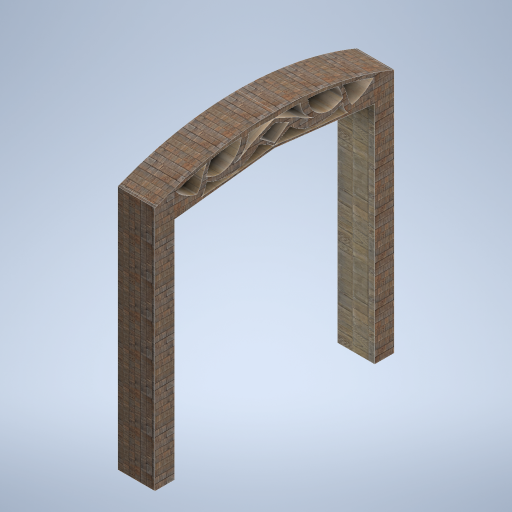
# Autodesk Inventor part: side_door_frame
Saved by Autodesk Inventor 2024.2 (Build 282272000, 272)
## iProperties
Created: 2024-05-27
Part Number: side_door_frame
Material: Wood (Maple)
Document SubType Name: Modeling
Designer: LOSTER_1
Density: 0.67 g/cm^3
Appearance: Natural Maple - Glossy Dark Tint
Author: LOSTER_1
Autodesk Inventor part; units mm, degrees
ref_plane "YZ Plane" through (0, 0, 0) normal (1, 0, 0) x (0, 1, 0)
ref_plane "XZ Plane" through (0, 0, 0) normal (0, 1, 0) x (-1, 0, 0)
ref_plane "XY Plane" through (0, 0, 0) normal (0, 0, 1) x (1, 0, 0)
sketch "Sketch1" plane through (0, 0, 0) normal (1, 0, 0) x (0, 1, 0)
  arc A0 (1227.0996, 1213.6257) -> (1219.0039, 1233.4807) centre (-1740.0857, 15.3721) ccw
  arc A1 (1293.746, 1033.6257) -> (1227.0996, 1213.6257) centre (-1739.133, 13.0159) ccw
  arc A2 (1300.346, 1013.7992) -> (1293.746, 1033.6257) centre (-1739.133, 13.0159) ccw
  arc A3 (1353.8129, 833.7992) -> (1300.346, 1013.7992) centre (-1739.133, 13.0159) ccw
  arc A4 (1359.0618, 813.7583) -> (1353.8129, 833.7992) centre (-1739.133, 13.0159) ccw
  arc A5 (1400.0832, 633.7583) -> (1359.0618, 813.7583) centre (-1739.133, 13.0159) ccw
  arc A6 (1403.9797, 613.7174) -> (1400.0832, 633.7583) centre (-1739.133, 13.0159) ccw
  arc A7 (1433.0918, 433.7174) -> (1403.9797, 613.7174) centre (-1739.133, 13.0159) ccw
  arc A8 (1453.264, 233.4731) -> (1435.7109, 413.4731) centre (-1739.133, 13.0159) ccw
  arc A9 (1435.7109, 413.4731) -> (1433.0918, 433.7174) centre (-1739.133, 13.0159) ccw
  arc A10 (1454.5841, 213.442) -> (1453.264, 233.4731) centre (-1739.133, 13.0159) ccw
  arc A11 (1460.8042, 33.0557) -> (1454.5841, 213.442) centre (-1739.133, 13.0159) ccw
  arc A12 (1460.867, 13.0444) -> (1460.8042, 33.0557) centre (-1739.133, 13.0159) ccw
  line L0 (-1280.9961, 1233.4807) -> (1219.0039, 1233.4807)
  line L1 (-1280.9961, 1233.4807) -> (-1280.9961, 1033.4807)
  line L2 (-1280.9961, 1033.4807) -> (1019.0039, 1033.4807)
  line L3 (1019.0039, 1033.4807) -> (1138.5556, 13.0444)
  line L4 (1460.867, 13.0444) -> (1469.3401, 13.0444)
  line L5 (1402.0541, 13.0444) -> (1293.7527, 249.1451)
  line L6 (1293.7527, 249.1451) -> (1163.5573, 13.0444)
  arc A13 (1208.0697, 415.2091) -> (1293.7527, 249.1451) centre (1799.1105, 615.028) ccw
  arc A14 (1232.0349, 708.2436) -> (1190.1135, 593.1028) centre (1522.2816, 537.3662) ccw
  arc A15 (1128.8881, 470.6135) -> (1251.1701, 171.9244) centre (1578.7407, 480.4058) ccw
  arc A16 (1191.7037, 709.8957) -> (1128.8881, 470.6135) centre (1578.7407, 480.4058) ccw
  arc A17 (1042.3948, 833.8278) -> (1191.7037, 709.8957) centre (1193.4877, 863.9522) ccw
  arc A18 (1400.0832, 633.7583) -> (1232.0349, 708.2436) centre (1155.9138, 309.6924) ccw
  arc A19 (1390.4476, 680.6424) -> (1228.9697, 753.7281) centre (1125.8269, 310.9107) ccw
  arc A20 (1190.1135, 593.1028) -> (1442.5544, 354.8708) centre (1416.5041, 580.1314) ccw
  arc A21 (1208.0697, 415.2091) -> (1449.7856, 279.0945) centre (1417.3067, 504.0976) ccw
  arc A22 (1290.1375, 1044.287) -> (1125.8335, 802.5328) centre (1497.6402, 726.5511) ccw
  arc A23 (1260.8526, 1126.6075) -> (1078.7798, 848.8845) centre (1573.2668, 723.2474) ccw
  arc A24 (1028.8129, 949.7563) -> (1078.7798, 848.8845) centre (1290.1521, 1016.3994) ccw
  arc A25 (1125.8335, 802.5328) -> (1228.9697, 753.7281) centre (1290.1521, 1016.3994) ccw
  line L7 (1359.0618, 13.0444) -> (1293.7527, 162.4218)
  line L8 (1293.7527, 162.4218) -> (1183.7754, 13.0444)
  line L9 (1460.867, 13.0444) -> (1635.1821, 13.0444)
  arc A26 (1219.0039, -1207.3919) -> (1227.0996, -1187.5369) centre (-1740.0857, 10.7167) ccw
  arc A27 (1227.0996, -1187.5369) -> (1293.746, -1007.5369) centre (-1739.133, 13.073) ccw
  arc A28 (1293.746, -1007.5369) -> (1300.346, -987.7104) centre (-1739.133, 13.073) ccw
  arc A29 (1300.346, -987.7104) -> (1353.8129, -807.7104) centre (-1739.133, 13.073) ccw
  arc A30 (1353.8129, -807.7104) -> (1359.0618, -787.6695) centre (-1739.133, 13.073) ccw
  arc A31 (1359.0618, -787.6695) -> (1400.0832, -607.6695) centre (-1739.133, 13.073) ccw
  arc A32 (1400.0832, -607.6695) -> (1403.9797, -587.6286) centre (-1739.133, 13.073) ccw
  arc A33 (1403.9797, -587.6286) -> (1433.0918, -407.6286) centre (-1739.133, 13.073) ccw
  arc A34 (1435.7109, -387.3843) -> (1453.264, -207.3843) centre (-1739.133, 13.073) ccw
  arc A35 (1433.0918, -407.6286) -> (1435.7109, -387.3843) centre (-1739.133, 13.073) ccw
  arc A36 (1453.264, -207.3843) -> (1454.5841, -187.3532) centre (-1739.133, 13.073) ccw
  arc A37 (1454.5841, -187.3532) -> (1460.8042, -6.9669) centre (-1739.133, 13.073) ccw
  arc A38 (1460.8042, -6.9669) -> (1460.867, 13.0444) centre (-1739.133, 13.073) ccw
  line L10 (-1280.9961, -1207.3919) -> (1219.0039, -1207.3919)
  line L11 (-1280.9961, -1207.3919) -> (-1280.9961, -1007.3919)
  line L12 (-1280.9961, -1007.3919) -> (1019.0039, -1007.3919)
  line L13 (1019.0039, -1007.3919) -> (1138.5556, 13.0444)
  line L14 (1402.0541, 13.0444) -> (1293.7527, -223.0563)
  line L15 (1293.7527, -223.0563) -> (1163.5573, 13.0444)
  arc A39 (1293.7527, -223.0563) -> (1208.0697, -389.1203) centre (1799.1105, -588.9392) ccw
  arc A40 (1190.1135, -567.014) -> (1232.0349, -682.1547) centre (1522.2816, -511.2774) ccw
  arc A41 (1251.1701, -145.8356) -> (1128.8881, -444.5247) centre (1578.7407, -454.317) ccw
  arc A42 (1128.8881, -444.5247) -> (1191.7037, -683.8069) centre (1578.7407, -454.317) ccw
  arc A43 (1191.7037, -683.8069) -> (1042.3948, -807.7389) centre (1193.4877, -837.8633) ccw
  arc A44 (1232.0349, -682.1547) -> (1400.0832, -607.6695) centre (1155.9138, -283.6036) ccw
  arc A45 (1228.9697, -727.6392) -> (1390.4476, -654.5536) centre (1125.8269, -284.8219) ccw
  arc A46 (1442.5544, -328.782) -> (1190.1135, -567.014) centre (1416.5041, -554.0426) ccw
  arc A47 (1449.7856, -253.0056) -> (1208.0697, -389.1203) centre (1417.3067, -478.0088) ccw
  arc A48 (1125.8335, -776.444) -> (1290.1375, -1018.1981) centre (1497.6402, -700.4623) ccw
  arc A49 (1078.7798, -822.7957) -> (1260.8526, -1100.5187) centre (1573.2668, -697.1585) ccw
  arc A50 (1078.7798, -822.7957) -> (1028.8129, -923.6674) centre (1290.1521, -990.3106) ccw
  arc A51 (1228.9697, -727.6392) -> (1125.8335, -776.444) centre (1290.1521, -990.3106) ccw
  line L16 (1359.0618, 13.0444) -> (1293.7527, -136.333)
  line L17 (1293.7527, -136.333) -> (1183.7754, 13.0444)
  arc A52 (1078.7798, 761.0996) -> (1163.5573, 13.0444) centre (10853.7042, 1490.0655) ccw
  arc A53 (1347.9034, 707.6571) -> (1256.4763, 1019.5586) centre (-1233.1421, 120.4308) ccw
  arc A54 (1403.56, 353.7392) -> (1357.9586, 661.5664) centre (7.3802, 304.2011) ccw
  arc A55 (1402.0541, 13.0444) -> (1404.1764, 277.1419) centre (-1314.3487, 166.9313) ccw
  arc A56 (1163.5573, 13.0444) -> (1078.7798, -735.0108) centre (10853.7042, -1463.9767) ccw
  arc A57 (1256.4763, -993.4698) -> (1347.9034, -681.5682) centre (-1233.1421, -94.3419) ccw
  arc A58 (1357.9586, -635.4776) -> (1403.56, -327.6504) centre (7.3802, -278.1123) ccw
  arc A59 (1404.1764, -251.0531) -> (1402.0541, 13.0444) centre (-1314.3487, -140.8425) ccw
  point P0 (0, 0)
  point P1 (1183.7754, 13.0444)
  point P2 (1359.0618, 13.0444)
  point P3 (1402.0541, 13.0444)
  point P4 (1163.5573, 13.0444)
  point P5 (1078.7798, -735.0108)
  point P6 (1163.5573, 13.0444)
  point P7 (1138.5556, 13.0444)
  point P8 (1347.9034, -681.5682)
  point P9 (1256.4763, -993.4698)
  point P10 (1403.56, -327.6504)
  point P11 (1402.0541, 13.0444)
  point P12 (1404.1764, -251.0531)
  dimension "d0" = 200
  dimension "d1" = 2300
  constraints: 145 point on circle, 80 symmetric about line, 60 centre point, 36 end point, 6 coincident, 6 point on line, 1 concentric, 1 horizontal, 1 perpendicular, 30 other
  measures "d0" distance of L0.start L1.end
  measures "d1" distance of L1.end L2.end
extrude "Extrusion1" add sketch "Sketch1" along normal blind 380 contours A1 A23 A24 L3 L2 L1 L0 A0 | A1 A22 A25 A19 A5 A18 A14 A20 A8 A21 A13 L6 A15 A16 A17 L3 A24 A23 | A1 A2 A3 A4 A5 A19 A53 A22 | A17 A52 A56 A43 L13 L3 | A6 A7 A9 A8 A20 A54 A18 | A43 A42 A41 L15 A39 A47 A34 A46 A40 A44 A31 A45 A51 A48 A27 A49 A50 L13 | L6 L5 L14 L15 | A50 A49 A27 A26 L10 L11 L12 L13 | A55 A21 A8 A10 A11 A12 A38 A37 A36 A34 A47 A59 | A48 A57 A45 A31 A30 A29 A28 A27 | A34 A35 A33 A32 A44 A58 A46
body "Solid1"
